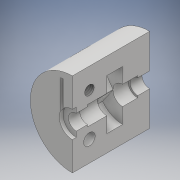
# Autodesk Inventor part: HalfEncoderSupprt
Saved by Autodesk Inventor 2018 (Build 220112000, 112)
## iProperties
Created: 2019-06-17
Part Number: HalfEncoderSupprt
Material: Generic
Document SubType Name: Modeling
Designer: aal_9
Density: 1 g/cm^3
Appearance: Default
Mass: 3.27571 g
Surface Area: 17.9664 cm^2
Volume: 3.27571 cm^3
Author: aal_9
Autodesk Inventor part; units mm, degrees
ref_plane "YZ Plane" through (0, 0, 0) normal (1, 0, 0) x (0, 1, 0)
ref_plane "XZ Plane" through (0, 0, 0) normal (0, 1, 0) x (-1, 0, 0)
ref_plane "XY Plane" through (0, 0, 0) normal (0, 0, 1) x (1, 0, 0)
sketch "Sketch1" plane through (0, 0, 0) normal (0, 1, 0) x (-1, 0, 0)
  arc A0 (0, -10.875) -> (0, 10.875) centre (0, 0) ccw
  line L0 (0, -10.875) -> (0, 10.875)
  dimension "d0" = 21.75
  constraints: 2 end point, 2 point on circle, 1 centre point, 1 coincident, 1 vertical
  measures "d0" diameter of A0
extrude "Extrusion1" add sketch "Sketch1" along normal blind 20
sketch "Sketch2" plane through (0, 20, 0) normal (0, 1, 0) x (1, 0, 0)
  circle A0 centre (0, 0) radius 2
  dimension "d3" = 4
  constraints: 1 centre point, 1 coincident
  measures "d3" diameter of A0
extrude "Extrusion2" cut sketch "Sketch2" against normal through all
ref_plane "Work Plane1" through (0, 13, 0) normal (0, -1, 0) x (1, 0, 0)
sketch "Sketch3" plane through (0, 13, 0) normal (0, -1, 0) x (1, 0, 0)
  line L0 (-2, -7.5208) -> (2, -7.5208) construction
  line L1 (2, -7.5208) -> (2, 8.0151) construction
  line L2 (2, 8.0151) -> (-2, 8.0151) construction
  line L3 (-2, 8.0151) -> (-2, -7.5208) construction
  line L4 (2.6754, -7.3078) -> (5.9521, -5.0135) construction
  line L5 (5.9521, -5.0135) -> (-2.959, 7.7128) construction
  line L6 (-2.959, 7.7128) -> (-6.2356, 5.4185) construction
  line L7 (-6.2356, 5.4185) -> (2.6754, -7.3078) construction
  line L8 (5.9521, 5.0135) -> (2.6754, 7.3078) construction
  line L9 (2.6754, 7.3078) -> (-6.2356, -5.4185) construction
  line L10 (-6.2356, -5.4185) -> (-2.959, -7.7128) construction
  line L11 (-2.959, -7.7128) -> (5.9521, 5.0135) construction
  line L12 (-5.1857, 3.919) -> (-2.4415, 0)
  line L13 (-5.1857, -3.919) -> (-2.4415, 0)
  line L14 (0, 10.875) -> (0, 2) projected
  line L15 (0, 6.4375) -> (0, -6.5)
  arc A0 (1.9091, -6.2133) -> (2, -6.1847) centre (0, 0) ccw
  arc A1 (2, 6.1847) -> (1.9091, 6.2133) centre (0, 0) ccw
  arc A2 (0, 6.5) -> (-5.1857, 3.919) centre (0, 0) ccw
  arc A3 (-5.1857, -3.919) -> (0, -6.5) centre (0, 0) ccw
  point P0 (2, 7.5208)
  point P1 (-2, -8.0151)
  dimension "d29" = 4
  dimension "d32" = 35
  dimension "d36" = 145
  constraints: 30 end point, 9 point on line, 8 point on circle, 4 centre point, 2 coincident, 2 parallel, 2 perpendicular, 1 collinear, 1 horizontal, 1 midpoint, 21 other
  measures "d29" distance of L2.end L1.end
extrude "Extrusion3" cut sketch "Sketch3" along normal blind 4.1
sketch "Sketch4" plane through (0, 20, 0) normal (0, 1, 0) x (1, 0, 0)
  line L0 (0, 0) -> (-10.2573, 10.2573) construction
  line L1 (0, 0) -> (14.5061, 0) construction
  point P0 (-5.1265, 5.1265)
  dimension "d38" = 7.25
  dimension "d39" = 225
  constraints: 4 end point, 1 equal length, 1 horizontal, 1 point on line
  measures "d38" distance of L0.start point (-5.127, 5.127)
hole "Hole1" at (-5.1265, 20, -5.1265) direction (0, -1, 0) diameter 1.567 depth 5 tip angle 118 thread size "M2x0.4" class "6H" standard "ISO Metric profile"
sketch "Sketch5" plane through (0, 0, 10.875) normal (1, 0, 0) x (0, 0, -1)
  line L0 (8.875, 8.9) -> (4.375, 8.9) projected
  line L1 (8.875, 0) -> (8.875, 8.9) projected
  point P0 (10.875, 0)
  point P1 (5.375, 4.4)
  dimension "d47" = 4.5
  dimension "d50" = 3.5
  measures "d47" distance from line of L0 point (5.375, 4.4)
  measures "d50" distance from line of L1 point (5.375, 4.4)
hole "Hole2" at (0, 4.4, 5.5) direction (-1, 0, 0) diameter 2.459 depth 5 tip angle 118 thread size "M3x0.5" class "6H" standard "ISO Metric profile"
sketch "Sketch6" plane through (0, 0, -10.875) normal (1, 0, 0) x (0, 0, -1)
  line L0 (-8.875, 8.9) -> (-8.875, 0) projected
  line L1 (-4.375, 8.9) -> (-8.875, 8.9) projected
  point P0 (-10.875, 0)
  point P1 (-5.375, 4.4)
  dimension "d58" = 3.5
  dimension "d59" = 4.5
  measures "d58" distance from line of point (-5.375, 4.4) L0
  measures "d59" distance from line of point (-5.375, 4.4) L1
hole "Hole3" at (0, 4.4, -5.5) direction (-1, 0, 0) diameter 3 end through all
ref_plane "Work Plane2" through (-11, 0, -10.875) normal (1, 0, 0) x (0, 0, -1)
sketch "Sketch7" plane through (-11, 0, -10.875) normal (1, 0, 0) x (0, 0, -1)
  circle A0 centre (-5.375, 4.4) radius 1.5 projected
  point P0 (-10.875, 0)
  constraints: 1 coincident
hole "Hole4" at (-11, 4.4, -5.5) direction (1, 0, 0) diameter 3 end through all counterbore diameter 4 counterbore depth 6
sketch "Sketch8" plane through (0, 0, 0) normal (0, -1, 0) x (1, 0, 0)
  circle A0 centre (0, 0) radius 2.7 construction
  line L0 (0, 3) -> (0, 2.4) construction
  line L1 (0, 6.5) -> (0, 2) projected
  arc A1 (-3, 1.6) -> (-3, -1.6) centre (0, 0) ccw
  arc A2 (-2.4, -2.4083) -> (-1.6, 3) centre (0, 0) ccw
  line L2 (-2.4, 9) -> (-3, 9)
  line L3 (-3, 9) -> (-3, 1.6)
  arc A3 (-3, 1.6) -> (-2.4, 2.4083) centre (0, 0) ccw
  arc A4 (-2.4, -2.4083) -> (-2.4, 2.4083) centre (0, 0) ccw
  arc A5 (-3, 1.6) -> (-3, -1.6) centre (0, 0) ccw
  line L4 (-2.4, 2.4083) -> (-2.4, 9)
  point P0 (0, 2.7)
  dimension "d76" = 5.4
  dimension "d80" = 0
  dimension "d88" = 0.6
  dimension "d89" = 9
  constraints: 12 point on circle, 8 end point, 5 centre point, 4 coincident, 1 parallel, 1 point on line, 1 vertical alignment, 2 other
  measures "d80" distance between parallel lines of L1 L0
  measures "d88" distance of L2.end L2.start
  measures "d89" distance from line of point (0, 0) L2
extrude "Extrusion4" cut sketch "Sketch8" against normal blind 1
sketch "Sketch9" plane through (0, 8.9, 0) normal (0, 1, 0) x (1, 0, 0)
  circle A0 centre (0, 0) radius 2.5
  dimension "d90" = 5
  constraints: 1 centre point, 1 coincident
  measures "d90" diameter of A0
extrude "Extrusion5" cut sketch "Sketch9" against normal blind 5 and the other way blind 8
sketch "Sketch10" plane through (0, 0, 0) normal (0, 0, 1) x (1, 0, 0)
  line L0 (-10.875, 0) -> (-10.875, 20) projected
  line L1 (-10.875, 12.5) -> (-7.875, 12.5)
  line L2 (-7.875, 12.5) -> (-7.875, 7.5)
  line L3 (-7.875, 7.5) -> (-10.875, 7.5)
  line L4 (-10.875, 7.5) -> (-10.875, 12.5)
  line L5 (0, 20) -> (-10.875, 20) projected
  point P0 (0, 0)
  dimension "d95" = 3
  dimension "d96" = 7.5
  dimension "d97" = 5
  constraints: 8 end point, 2 parallel, 1 horizontal, 1 perpendicular, 1 point on line
  measures "d95" distance of L2.end L3.end
  measures "d96" distance between parallel lines of L5 L1
  measures "d97" distance of L1.end L2.end
extrude "Extrusion6" cut sketch "Sketch10" along normal through all both and the other way through all
body "Solid1"
